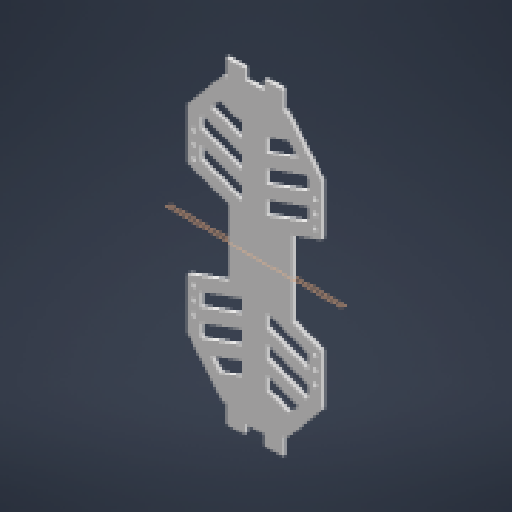
# Autodesk Inventor part: Backplane
Saved by Autodesk Inventor 2026.1 (Build 301233020, 233B)
## iProperties
Created: 2025-10-02
Part Number: Backplane
Material: Generic
Document SubType Name: Modeling
Designer: Malthe Sennels
Density: 1 g/cm^3
Appearance: Default
Author: Malthe Sennels
Autodesk Inventor part; units mm, degrees
ref_plane "YZ Plane" through (0, 0, 0) normal (1, 0, 0) x (0, 1, 0)
ref_plane "XZ Plane" through (0, 0, 0) normal (0, 1, 0) x (-1, 0, 0)
ref_plane "XY Plane" through (0, 0, 0) normal (0, 0, 1) x (1, 0, 0)
sketch "Sketch1" plane through (0, 0, 0) normal (0, 0, 1) x (1, 0, 0)
  line L0 (0, -13.8137) -> (15, -13.8137) projected
  line L1 (0, 0) -> (0, -13.8137) projected
  line L2 (45, 0) -> (0, 0) projected
  line L3 (45, 0) -> (45, -13.8137) projected
  line L4 (30, -13.8137) -> (45, -13.8137) projected
  line L5 (30, -6) -> (30, -13.8137) projected
  line L6 (30, -6) -> (15, -6) projected
  line L7 (15, -6) -> (15, -13.8137) projected
  line L8 (-2.5, 0) -> (-2.5, -11.3137) projected
  line L9 (47.5, 0) -> (-2.5, 0) projected
  line L10 (47.5, 0) -> (75, 32.7732)
  line L11 (47.5, 0) -> (90.2824, 0) construction
  line L12 (75, 32.7732) -> (75, 72.7732)
  line L13 (75, 72.7732) -> (52.5, 80.9626)
  line L14 (52.5, 80.9626) -> (52.5, 110.5752)
  line L15 (22.5, -6) -> (22.5, 110.5752)
  line L16 (-10.9317, 221.1504) -> (1.7683, 221.1504) construction
  line L17 (22.5, 0) -> (22.5, 221.1504)
  line L18 (22.5, 110.5752) -> (52.5, 110.5752) construction
  line L19 (-2.5, 0) -> (-30, 32.7732)
  line L20 (-30, 32.7732) -> (-30, 72.7732)
  line L21 (-30, 72.7732) -> (-7.5, 80.9626)
  line L22 (-7.5, 80.9626) -> (2.5, 84.6023)
  line L23 (2.5, 84.6023) -> (2.5, 110.5752)
  line L24 (22.5, 110.5752) -> (2.5, 110.5752) construction
  line L25 (47.5, 221.1504) -> (75, 188.3772)
  line L26 (75, 188.3772) -> (75, 148.3772)
  line L27 (75, 148.3772) -> (52.5, 140.1879)
  line L28 (52.5, 140.1879) -> (52.5, 110.5752)
  line L29 (-30, 148.3772) -> (-7.5, 140.1879)
  line L30 (-30, 188.3772) -> (-30, 148.3772)
  line L31 (-2.5, 221.1504) -> (-30, 188.3772)
  line L32 (-7.5, 140.1879) -> (2.5, 136.5482)
  line L33 (2.5, 136.5482) -> (2.5, 110.5752)
  line L34 (0, 234.9641) -> (15, 234.9641)
  line L35 (0, 221.1504) -> (0, 234.9641)
  line L36 (45, 221.1504) -> (45, 234.9641)
  line L37 (30, 234.9641) -> (45, 234.9641)
  line L38 (30, 227.1504) -> (30, 234.9641)
  line L39 (30, 227.1504) -> (15, 227.1504)
  line L40 (15, 227.1504) -> (15, 234.9641)
  line L41 (47.5, 221.1504) -> (-2.5, 221.1504)
  line L42 (75, 40) -> (75, 44.6908)
  dimension "d0" = 50
  dimension "d1" = 110
  dimension "d2" = 30
  dimension "d3" = 40
  dimension "d4" = 30
  dimension "d5" = 20
  constraints: 64 end point, 20 symmetric about line, 4 vertical, 3 horizontal, 3 midpoint, 3 point on line, 1 collinear, 1 equal length, 1 parallel, 1 perpendicular
  measures "d0" angle of L11 L10
  measures "d1" angle of L13 L12
  measures "d2" distance between parallel lines of L15 L14
  measures "d3" distance of L10.end L12.end
  measures "d4" horizontal distance of L2.start L10.end
  measures "d5" distance between parallel lines of L23 L15
extrude "Extrusion1" add sketch "Sketch1" along normal blind 3
sketch "Sketch2" plane through (0, 0, 3) normal (0, 0, 1) x (1, 0, 0)
  line L0 (45, -13.8137) -> (45, 0) projected
  line L1 (45, 0) -> (47.5, 0) projected
  line L2 (47.5, 0) -> (75, 32.7732) projected
  line L3 (75, 32.7732) -> (75, 72.7732) projected
  line L4 (75, 72.7732) -> (52.5, 80.9626) projected
  line L5 (52.5, 80.9626) -> (52.5, 140.1879) projected
  line L6 (52.5, 140.1879) -> (75, 148.3772) projected
  line L7 (75, 148.3772) -> (75, 188.3772) projected
  line L8 (75, 188.3772) -> (47.5, 221.1504) projected
  line L9 (47.5, 221.1504) -> (45, 221.1504) projected
  line L10 (45, 221.1504) -> (45, 234.9641) projected
  line L11 (45, 234.9641) -> (30, 234.9641) projected
  line L12 (30, 234.9641) -> (30, 227.1504) projected
  line L13 (30, 227.1504) -> (15, 227.1504) projected
  line L14 (15, 227.1504) -> (15, 234.9641) projected
  line L15 (15, 234.9641) -> (0, 234.9641) projected
  line L16 (0, 234.9641) -> (0, 221.1504) projected
  line L17 (0, 221.1504) -> (-2.5, 221.1504) projected
  line L18 (-2.5, 221.1504) -> (-30, 188.3772) projected
  line L19 (-30, 188.3772) -> (-30, 148.3772) projected
  line L20 (-30, 148.3772) -> (2.5, 136.5482) projected
  line L21 (2.5, 136.5482) -> (2.5, 84.6023) projected
  line L22 (2.5, 84.6023) -> (-30, 72.7732) projected
  line L23 (-30, 72.7732) -> (-30, 32.7732) projected
  line L24 (-30, 32.7732) -> (-2.5, 0) projected
  line L25 (-2.5, 0) -> (0, 0) projected
  line L26 (0, 0) -> (0, -13.8137) projected
  line L27 (0, -13.8137) -> (15, -13.8137) projected
  line L28 (15, -13.8137) -> (15, -6) projected
  line L29 (15, -6) -> (30, -6) projected
  line L30 (30, -6) -> (30, -13.8137) projected
  line L31 (30, -13.8137) -> (45, -13.8137) projected
  line L32 (-20, 36.4129) -> (-20, 65.7711)
  line L33 (-20, 65.7711) -> (12.5, 77.6002)
  line L34 (12.5, 77.6002) -> (12.5, 143.5503)
  line L35 (12.5, 143.5503) -> (-20, 155.3793)
  line L36 (-20, 155.3793) -> (-20, 184.7375)
  line L37 (-20, 184.7375) -> (2.1631, 211.1504)
  line L38 (2.1631, 211.1504) -> (10, 211.1504)
  line L39 (10, 211.1504) -> (10, 217.1504)
  line L40 (10, 217.1504) -> (35, 217.1504)
  line L41 (35, 217.1504) -> (35, 211.1504)
  line L42 (35, 211.1504) -> (42.8369, 211.1504)
  line L43 (42.8369, 211.1504) -> (65, 184.7375)
  line L44 (65, 184.7375) -> (65, 155.3793)
  line L45 (65, 155.3793) -> (42.5, 147.19)
  line L46 (42.5, 147.19) -> (42.5, 73.9605)
  line L47 (42.5, 73.9605) -> (65, 65.7711)
  line L48 (65, 65.7711) -> (65, 36.4129)
  line L49 (65, 36.4129) -> (42.8369, 10)
  line L50 (42.8369, 10) -> (35, 10)
  line L51 (35, 10) -> (35, 4)
  line L52 (35, 4) -> (10, 4)
  line L53 (10, 4) -> (10, 10)
  line L54 (10, 10) -> (2.1631, 10)
  line L55 (2.1631, 10) -> (-20, 36.4129)
  line L56 (12.5, 77.6002) -> (12.5, 10)
  line L57 (12.5, 10) -> (10, 10)
  line L58 (22.5, 4) -> (22.5, 217.1504) construction
  line L59 (32.5, 77.6002) -> (32.5, 10)
  line L60 (32.5, 10) -> (35, 10)
  line L61 (32.5, 77.6002) -> (32.5, 211.1504)
  line L62 (32.5, 211.1504) -> (35, 211.1504)
  line L63 (12.5, 143.5503) -> (12.5, 211.1504)
  line L64 (12.5, 211.1504) -> (10, 211.1504)
  line L65 (-20, 55.1294) -> (12.5, 66.9584)
  line L66 (-25.1903, 42.5985) -> (12.5, 56.3166)
  line L67 (-18.3499, 34.4464) -> (12.5, 45.6748)
  line L68 (-11.5095, 26.2943) -> (12.5, 35.0331)
  line L69 (-4.6691, 18.1423) -> (12.5, 24.3913)
  line L70 (65, 55.1294) -> (32.5, 66.9584)
  line L71 (70.1903, 42.5985) -> (32.5, 56.3166)
  line L72 (63.3499, 34.4464) -> (32.5, 45.6748)
  line L73 (56.5095, 26.2943) -> (32.5, 35.0331)
  line L74 (49.6691, 18.1423) -> (32.5, 24.3913)
  line L75 (42.5, 73.9605) -> (32.5, 77.6002)
  point P0 (32.5, 66.9584)
  point P1 (65, 55.1294)
  point P2 (73.2901, 46.2927)
  point P3 (32.5, 56.3166)
  point P4 (32.5, 45.6748)
  point P5 (63.3499, 34.4464)
  point P6 (56.5095, 26.2943)
  point P7 (32.5, 35.0331)
  point P8 (32.5, 24.3913)
  point P9 (49.6691, 18.1423)
  point P10 (65, 44.4876)
  point P11 (-20, 44.4876)
  dimension "d8" = 10
  dimension "d9" = 10
  dimension "d10" = 10
  dimension "d11" = 10
  dimension "d12" = 10
  dimension "d13" = 10
  constraints: 88 end point, 12 symmetric about line, 10 point on line, 5 parallel, 4 perpendicular, 2 midpoint, 2 vertical, 23 other
  measures "d8" distance between parallel lines of L23 L32
  measures "d9" distance between parallel lines of L65 L33
  measures "d10" distance between parallel lines of L65 L66
  measures "d11" distance between parallel lines of L66 L67
  measures "d12" distance between parallel lines of L67 L68
  measures "d13" distance between parallel lines of L68 L69
extrude "Extrusion2" cut sketch "Sketch2" against normal blind 3 contours L32 L33 L56 L65 | L66 L56 L67 L55 L32 | L68 L56 L69 L55 | L75 L47 L48 L70 L59 | L71 L48 L49 L72 L59 | L74 L59 L73 L49
ref_plane "Work Plane1" through (0, 110.5752, 0) normal (0, 1, 0) x (1, 0, 0)
mirror "Mirror1" about plane through (0, 110.5752, 0) normal (0, 1, 0) of "Extrusion2"
sketch "Sketch3" plane through (0, 0, 0) normal (0, 0, -1) x (-1, 0, 0)
  line L0 (4.6691, 203.0082) -> (11.5095, 194.8561) projected
  line L1 (-32.5, 143.5503) -> (-65, 155.3793) projected
  line L2 (-65, 155.3793) -> (-65, 166.0211) projected
  line L3 (-56.5095, 194.8561) -> (-49.6691, 203.0082) projected
  line L4 (20, 166.0211) -> (20, 155.3793) projected
  line L5 (20, 155.3793) -> (-12.5, 143.5503) projected
  line L6 (11.5095, 26.2943) -> (4.6691, 18.1423) projected
  line L7 (-65, 55.1294) -> (-65, 65.7711) projected
  line L8 (-65, 65.7711) -> (-32.5, 77.6002) projected
  line L9 (-49.6691, 18.1423) -> (-56.5095, 26.2943) projected
  line L10 (-12.5, 77.6002) -> (20, 65.7711) projected
  line L11 (20, 65.7711) -> (20, 55.1294) projected
  line L12 (-45, -13.8137) -> (-45, 0) projected
  line L13 (-30, -13.8137) -> (-45, -13.8137) projected
  line L14 (-30, -6) -> (-30, -13.8137) projected
  line L15 (-15, -6) -> (-30, -6) projected
  line L16 (-15, -13.8137) -> (-15, -6) projected
  line L17 (0, -13.8137) -> (-15, -13.8137) projected
  line L18 (0, 0) -> (0, -13.8137) projected
  line L19 (2.5, 0) -> (0, 0) projected
  line L20 (30, 32.7732) -> (2.5, 0) projected
  line L21 (30, 72.7732) -> (30, 32.7732) projected
  line L22 (-2.5, 84.6023) -> (30, 72.7732) projected
  line L23 (-2.5, 136.5482) -> (-2.5, 84.6023) projected
  line L24 (30, 148.3772) -> (-2.5, 136.5482) projected
  line L25 (30, 188.3772) -> (30, 148.3772) projected
  line L26 (2.5, 221.1504) -> (30, 188.3772) projected
  line L27 (0, 221.1504) -> (2.5, 221.1504) projected
  line L28 (0, 234.9641) -> (0, 221.1504) projected
  line L29 (-15, 234.9641) -> (0, 234.9641) projected
  line L30 (-15, 227.1504) -> (-15, 234.9641) projected
  line L31 (-30, 227.1504) -> (-15, 227.1504) projected
  line L32 (-30, 234.9641) -> (-30, 227.1504) projected
  line L33 (-45, 234.9641) -> (-30, 234.9641) projected
  line L34 (-45, 221.1504) -> (-45, 234.9641) projected
  line L35 (-47.5, 221.1504) -> (-45, 221.1504) projected
  line L36 (-75, 188.3772) -> (-47.5, 221.1504) projected
  line L37 (-75, 148.3772) -> (-75, 188.3772) projected
  line L38 (-52.5, 140.1879) -> (-75, 148.3772) projected
  line L39 (-52.5, 80.9626) -> (-52.5, 140.1879) projected
  line L40 (-75, 72.7732) -> (-52.5, 80.9626) projected
  line L41 (-75, 32.7732) -> (-75, 72.7732) projected
  line L42 (-47.5, 0) -> (-75, 32.7732) projected
  line L43 (-45, 0) -> (-47.5, 0) projected
  circle A0 centre (25, 67.7732) radius 1.75
  circle A1 centre (25, 57.7732) radius 1.75
  circle A2 centre (25, 47.7732) radius 1.75
  line L44 (-2.5, 136.5482) -> (-2.5, 84.6023) projected
  line L45 (-2.5, 110.5752) -> (-52.5, 110.5752)
  circle A3 centre (25, 153.3772) radius 1.75
  circle A4 centre (25, 163.3772) radius 1.75
  circle A5 centre (25, 173.3772) radius 1.75
  line L46 (-15, -6) -> (-30, -6) projected
  line L47 (-22.5, -6) -> (-22.5, 227.1504)
  line L48 (-30, 227.1504) -> (-15, 227.1504) projected
  circle A6 centre (-70, 67.7732) radius 1.75
  circle A7 centre (-70, 57.7732) radius 1.75
  circle A8 centre (-70, 47.7732) radius 1.75
  circle A9 centre (-70, 153.3772) radius 1.75
  circle A10 centre (-70, 163.3772) radius 1.75
  circle A11 centre (-70, 173.3772) radius 1.75
  line L49 (-12.5, 154.192) -> (20, 166.0211) projected
  line L50 (-12.5, 143.5503) -> (-12.5, 154.192) projected
  line L51 (-49.6691, 203.0082) -> (-32.5, 196.7591) projected
  line L52 (-32.5, 196.7591) -> (-32.5, 186.1174) projected
  line L53 (-32.5, 186.1174) -> (-56.5095, 194.8561) projected
  line L54 (-32.5, 154.192) -> (-32.5, 143.5503) projected
  line L55 (-65, 166.0211) -> (-32.5, 154.192) projected
  line L56 (11.5095, 194.8561) -> (-12.5, 186.1174) projected
  line L57 (-12.5, 186.1174) -> (-12.5, 196.7591) projected
  line L58 (-12.5, 196.7591) -> (4.6691, 203.0082) projected
  line L59 (20, 55.1294) -> (-12.5, 66.9584) projected
  line L60 (-12.5, 66.9584) -> (-12.5, 77.6002) projected
  line L61 (-32.5, 24.3913) -> (-49.6691, 18.1423) projected
  line L62 (-56.5095, 26.2943) -> (-32.5, 35.0331) projected
  line L63 (-32.5, 35.0331) -> (-32.5, 24.3913) projected
  line L64 (-32.5, 77.6002) -> (-32.5, 66.9584) projected
  line L65 (-32.5, 66.9584) -> (-65, 55.1294) projected
  line L66 (-12.5, 35.0331) -> (11.5095, 26.2943) projected
  line L67 (4.6691, 18.1423) -> (-12.5, 24.3913) projected
  line L68 (-12.5, 24.3913) -> (-12.5, 35.0331) projected
  dimension "d16" = 3.5
  dimension "d19" = 10
  dimension "d24" = 5
  dimension "d25" = 5
  constraints: 12 centre point, 9 symmetric about line, 4 end point, 4 midpoint, 1 vertical, 13 other
  measures "d16" diameter of A0
  measures "d19" distance of A0.centre A1.centre
  measures "d24" distance from line of L21 A0.centre
  measures "d25" horizontal distance of L21.start A0.centre
extrude "Extrusion3" cut sketch "Sketch3" against normal through all contours A0 | A1 | A2 | A3 | A4 | A5 | A6 | A7 | A8 | A9 | A10 | A11
body "Solid1"
